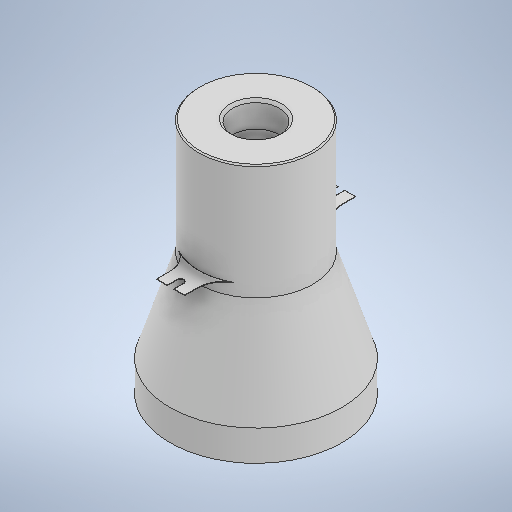
# Autodesk Inventor part: shaker
Saved by Autodesk Inventor 2025 (Build 290162000, 162)
## iProperties
Created: 2024-06-18
Part Number: shaker
Material: Generic
Document SubType Name: Modeling
Designer: mumin
Density: 1 g/cm^3
Appearance: Default
Author: mumin
Autodesk Inventor part; units mm, degrees
ref_plane "YZ Plane" through (0, 0, 0) normal (1, 0, 0) x (0, 1, 0)
ref_plane "XY Plane" through (0, 0, 0) normal (0, 0, 1) x (1, 0, 0)
sketch "Sketch1" plane through (0, 0, 0) normal (0, 1, 0) x (-1, 0, 0)
  circle A0 centre (0, 0) radius 22.4
  dimension "d0" = 44.8
  constraints: 1 centre point, 1 coincident
  measures "d0" diameter of A0
ref_plane "Work Plane1" through (0, 40.5, 0) normal (0, 1, 0) x (-1, 0, 0)
sketch "Sketch2" plane through (0, 40.5, 0) normal (0, 1, 0) x (-1, 0, 0)
  circle A0 centre (0, 0) radius 22.4 projected
ref_plane "Work Plane3" through (0, -53, 0) normal (0, 1, 0) x (-1, 0, 0)
ref_plane "Work Plane2" through (0, -41, 0) normal (0, 1, 0) x (-1, 0, 0)
sketch "Sketch3" plane through (0, -41, 0) normal (0, 1, 0) x (-1, 0, 0)
  circle A0 centre (0, 0) radius 33.8
  dimension "d4" = 67.6
  constraints: 1 centre point, 1 coincident
  measures "d4" diameter of A0
sketch "Sketch4" plane through (0, -53, 0) normal (0, 1, 0) x (-1, 0, 0)
  circle A0 centre (0, 0) radius 33.8 projected
loft "Loft1" add profiles "Sketch2", "Sketch1"
loft "Loft3" [suppressed]
sketch "Sketch5" plane through (0, 0, 0) normal (0, 1, 0) x (-1, 0, 0)
  line L0 (-5.5, 33.6) -> (5.5, -33.6) construction
  line L1 (3.6185, 22.1058) -> (-5.5, -33.6) construction
  line L2 (5.5, 33.6) -> (5.5, 28.4519)
  line L3 (5.5, -28.4519) -> (5.5, -33.6)
  line L4 (-5.5, -33.6) -> (-5.5, -28.4519)
  line L5 (-5.5, 28.4519) -> (-5.5, 33.6)
  arc A0 (-10.716, 19.6704) -> (-10.716, -19.6704) centre (0, 0) ccw
  arc A1 (10.716, -19.6704) -> (10.716, 19.6704) centre (0, 0) ccw
  arc A2 (5.5, 28.4519) -> (10.716, 19.6704) centre (15.5, 28.4519) ccw
  arc A3 (-10.716, 19.6704) -> (-5.5, 28.4519) centre (-15.5, 28.4519) ccw
  arc A4 (10.716, -19.6704) -> (5.5, -28.4519) centre (15.5, -28.4519) ccw
  arc A5 (-5.5, -28.4519) -> (-10.716, -19.6704) centre (-15.5, -28.4519) ccw
  circle A6 centre (0, 0) radius 22.4 construction
  line L6 (0, -22.4) -> (0, -33.6) construction
  line L7 (1.3, -33.6) -> (1.3, -29.7)
  line L8 (0, -28.4) -> (0, -28.4)
  line L9 (-1.3, -29.7) -> (-1.3, -33.6)
  arc A7 (1.3, -29.7) -> (0, -28.4) centre (0, -29.7) ccw
  arc A8 (0, -28.4) -> (-1.3, -29.7) centre (0, -29.7) ccw
  line L10 (5.5, -33.6) -> (1.3, -33.6)
  line L11 (-1.3, -33.6) -> (-5.5, -33.6)
  circle A9 centre (0, 0) radius 33.8 construction
  line L12 (33.8, 0) -> (-33.8, 0) construction
  line L13 (0, 22.4) -> (0, 33.6) construction
  line L14 (1.3, 33.6) -> (1.3, 29.7)
  line L15 (-1.3, 29.7) -> (-1.3, 33.6)
  arc A10 (0, 28.4) -> (1.3, 29.7) centre (0, 29.7) ccw
  arc A11 (-1.3, 29.7) -> (0, 28.4) centre (0, 29.7) ccw
  line L16 (5.5, 33.6) -> (1.3, 33.6)
  line L17 (-1.3, 33.6) -> (-5.5, 33.6)
  circle A12 centre (0, 0) radius 33.8 construction
  point P0 (5.5, 21.7143)
  point P1 (5.5, -21.7143)
  point P2 (-5.5, 21.7143)
  point P3 (-5.5, -21.7143)
  point P4 (1.3, -28.4)
  point P5 (-1.3, -28.4)
  point P6 (1.3, 28.4)
  point P7 (-1.3, 28.4)
  point P8 (0, 28.4)
  dimension "d17" = 11
  dimension "d18" = 67.2
  dimension "d19" = 10
  dimension "d20" = 2.6
  dimension "d21" = 5.2
  dimension "d22" = 1.3
  constraints: 36 end point, 26 point on circle, 12 symmetric about line, 12 tangent, 11 centre point, 11 point on line, 4 equal radius, 4 parallel, 2 perpendicular, 2 vertical, 1 coincident, 1 horizontal, 1 midpoint, 6 other
  measures "d17" distance of L0.end L1.end
  measures "d18" distance of L2.start L0.end
  measures "d19" radius of A2
  measures "d20" distance of point (1.3, -28.4) point (-1.3, -28.4)
  measures "d21" distance of L7.start point (1.3, -28.4)
  measures "d22" radius of A7
extrude "Extrusion1" add sketch "Sketch5" against normal blind 0.2
ref_plane "Work Plane4" through (0, -4.7, 0) normal (0, 1, 0) x (-1, 0, 0)
sketch "Sketch6" plane through (0, -4.7, 0) normal (0, 1, 0) x (-1, 0, 0)
  circle A0 centre (0, 0) radius 22.4 projected
ref_plane "Work Plane5" through (0, -53, 0) normal (0, 1, 0) x (-1, 0, 0)
sketch "Sketch7" plane through (0, -53, 0) normal (0, 1, 0) x (-1, 0, 0)
  circle A0 centre (0, 0) radius 33.8 projected
loft "Loft4" add profiles "Sketch7", "Sketch3"
loft "Loft5" add profiles "Sketch6" section 1 edges at (33.8, -41, 0)
sketch "Sketch8" plane through (0, 0, 0) normal (0, 1, 0) x (-1, 0, 0)
  circle A0 centre (0, 0) radius 22.4 projected
loft "Loft6" add profiles "Sketch8" section 2 edges at (22.4, -4.7, 0)
sketch "Sketch9" plane through (0, 40.5, 0) normal (0, 1, 0) x (1, 0, 0)
  point P0 (0, 0)
  point P1 (0, 0)
  constraints: 1 coincident
hole "Hole1" at (0, 40.5, 0) direction (0, -1, 0) diameter 18.4 depth 10
chamfer "Chamfer1" distance 1 angle 45 1 edges at (0, 40.5, -9.2)
chamfer "Chamfer2" distance 0.5 angle 45 1 edges at (22.4, 40.5, 0)
sketch "Sketch10" plane through (0, -53, 0) normal (0, -1, 0) x (1, 0, 0)
  point P0 (0, 0)
  point P1 (0, 0)
  constraints: 1 coincident
hole "Hole2" at (0, -53, 0) direction (0, 1, 0) diameter 13.5 depth 10
body "Solid1"
